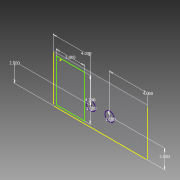
# Autodesk Inventor part: board
Saved by Autodesk Inventor 2015 (Build 190159000, 159)
## iProperties
Created: 2015-01-05
Part Number: board
Material: Acrylic, Clear
Document SubType Name: Modeling
Designer: techlab
Density: 1.19 g/cm^3
Appearance: Transparent - Clear
Author: techlab
Autodesk Inventor part; units mm, degrees
ref_plane "YZ Plane" through (0, 0, 0) normal (1, 0, 0) x (0, 1, 0)
ref_plane "XZ Plane" through (0, 0, 0) normal (0, 1, 0) x (-1, 0, 0)
ref_plane "XY Plane" through (0, 0, 0) normal (0, 0, 1) x (1, 0, 0)
sketch "Sketch1" plane through (0, 0, 0) normal (0, 0, 1) x (1, 0, 0)
  point P0 (0, 0)
sketch "Sketch2" plane through (0, 0, 0) normal (0, 0, 1) x (1, 0, 0)
  line L0 (-15.8604, 11.7809) -> (231.7896, 11.7809)
  line L1 (234.9646, 8.6059) -> (234.9646, -112.0441)
  line L2 (231.7896, -115.2191) -> (-15.8604, -115.2191)
  line L3 (-19.0354, -112.0441) -> (-19.0354, 8.6059)
  arc A0 (-15.8604, 11.7809) -> (-19.0354, 8.6059) centre (-15.8604, 8.6059) ccw
  arc A1 (234.9646, 8.6059) -> (231.7896, 11.7809) centre (231.7896, 8.6059) ccw
  arc A2 (231.7896, -115.2191) -> (234.9646, -112.0441) centre (231.7896, -112.0441) ccw
  arc A3 (-19.0354, -112.0441) -> (-15.8604, -115.2191) centre (-15.8604, -112.0441) ccw
  point P0 (0, 0)
  point P1 (234.9646, -115.2191)
  point P2 (234.9646, 11.7809)
  point P3 (-19.0354, -115.2191)
  dimension "d0" = 254
  dimension "d1" = 127
  dimension "d2" = 3.175
  constraints: 8 end point, 8 point on circle, 8 tangent, 6 point on line, 4 centre point, 3 equal radius, 2 parallel, 1 horizontal, 1 perpendicular
  measures "d0" distance of point (234.965, -115.219) point (-19.035, -115.219)
  measures "d1" distance of point (234.965, 11.781) point (234.965, -115.219)
  measures "d2" radius of A0
extrude "Extrusion1" add sketch "Sketch2" along normal blind 2.54
sketch "Sketch3" plane through (0, 0, 2.54) normal (0, 0, 1) x (1, 0, 0)
  circle A0 centre (82.5646, -64.4191) radius 12.7
  circle A1 centre (133.3646, -64.4191) radius 12.7
  line L0 (-19.0354, 8.6059) -> (-19.0354, -112.0441) projected
  line L1 (234.9646, -112.0441) -> (234.9646, 8.6059) projected
  line L2 (-15.8604, -115.2191) -> (231.7896, -115.2191) projected
  point P0 (0, 0)
  dimension "d5" = 25.4
  dimension "d6" = 25.4
  dimension "d7" = 101.6
  dimension "d8" = 101.6
  dimension "d9" = 50.8
  dimension "d10" = 50.8
  constraints: 2 centre point
  measures "d5" diameter of A0
  measures "d6" diameter of A1
  measures "d7" distance from line of L0 A0.centre
  measures "d8" distance from line of A1.centre L1
  measures "d9" distance from line of L2 A0.centre
  measures "d10" distance from line of L2 A1.centre
extrude "Extrusion2" cut sketch "Sketch3" against normal blind 50.8
sketch "Sketch4" plane through (0, 0, 2.54) normal (0, 0, 1) x (1, 0, 0)
  line L0 (-10.6768, -109.1793) -> (65.5232, -109.1793)
  line L1 (65.5232, -109.1793) -> (65.5232, 5.1207)
  line L2 (65.5232, 5.1207) -> (-10.6768, 5.1207)
  line L3 (-10.6768, 5.1207) -> (-10.6768, -109.1793)
  point P0 (0, 0)
  dimension "d13" = 76.2
  dimension "d14" = 114.3
  constraints: 8 end point, 2 parallel, 1 horizontal, 1 perpendicular
  measures "d13" distance of L2.end L1.end
  measures "d14" distance of L1.end L0.end
body "Solid1"
